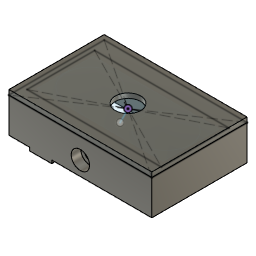
couvercle2_female (Autodesk Fusion 360 design; units mm, degrees)
Autodesk Fusion 360 part; units mm, degrees
sketch "Esquisse7" plane through (0, 0, 10) normal (0, 0, 1) x (-1, 0, 0)
  circle A0 centre (-12, 0) radius 7.6
  circle A1 centre (12, 0) radius 7.6
  line L0 (-19.9, -8.9) -> (19.9, -8.9)
  line L1 (19.9, -8.9) -> (19.9, 8.9)
  line L2 (19.9, 8.9) -> (-19.9, 8.9)
  line L3 (-19.9, 8.9) -> (-19.9, -8.9)
  line L4 (0, 0) -> (-2.53, 5.0152)
  constraint coincident L4.start origin
sketch "Esquisse3" plane through (0, 0, 10) normal (0, 0, 1) x (-1, 0, 0)
  line L0 (21.15, -10.65) -> (-21.15, -10.65)
  line L1 (-21.15, -10.65) -> (-21.15, 10.65)
  line L2 (-21.15, 10.65) -> (21.15, 10.65)
  line L3 (21.15, 10.65) -> (21.15, -10.65)
  line L4 (21.15, -10.65) -> (-21.15, 10.65) construction
  line L5 (-21.15, -10.65) -> (21.15, 10.65) construction
  line L6 (22.5, -15) -> (-22.5, -15)
  line L7 (-22.5, -15) -> (-22.5, 15)
  line L8 (-22.5, 15) -> (22.5, 15)
  line L9 (22.5, 15) -> (22.5, -15)
  line L10 (22.5, -15) -> (-22.5, 15) construction
  line L11 (-22.5, -15) -> (22.5, 15) construction
  dimension "d76" = 42.3
  dimension "d77" = 21.3
  dimension "d78" = 45
  dimension "d79" = 30
  constraint horizontal L0
  constraint perpendicular L0 L1
  constraint parallel L0 L2
  constraint parallel L1 L3
  constraint coincident L4 origin
  constraint coincident L5 origin
  constraint horizontal L6
  constraint perpendicular L6 L7
  constraint parallel L6 L8
  constraint parallel L7 L9
  constraint coincident L10 origin
  constraint coincident L11 origin
  measures "d76" distance of L1.end L2.end
  measures "d77" distance of L0.end L1.end
  measures "d78" distance of L7.end L8.end
  measures "d79" distance of L6.end L7.end
extrude "Extrusion1" add sketch "Esquisse3" against normal blind 11
extrude "Extrusion2" add sketch "Esquisse3" along normal blind 1.5 contours L0 L1 L2 L3 | L6 L7 L8 L9
sketch "Esquisse4" plane through (0, -15, 0) normal (0, -1, 0) x (1, 0, 0)
  line L0 (-22.5, 11.5) -> (-22.5, -1)
  line L1 (-22.5, -1) -> (22.5, -1)
  line L2 (22.5, -1) -> (22.5, 11.5)
  line L3 (22.5, 11.5) -> (-22.5, 11.5)
  line L4 (0, 0) -> (0, 3.5)
  dimension "d84" = 3.5
  constraint coincident L4.start origin
  constraint vertical L4
  measures "d84" distance of L4.start L4.end
hole "Perçage1" at (0, -15, 3.5) direction (0, 1, 0) diameter 3.3 depth 8 tip angle 180 counterbore diameter 5.8 counterbore depth 3
sketch "Esquisse5" plane through (0, 15, 0) normal (0, 1, 0) x (-1, 0, 0)
  line L0 (-22.5, 11.5) -> (-22.5, -1)
  line L1 (-22.5, -1) -> (22.5, -1)
  line L2 (22.5, -1) -> (22.5, 11.5)
  line L3 (22.5, 11.5) -> (-22.5, 11.5)
  line L4 (0, 0) -> (0, 3.5)
  dimension "d100" = 3.5
  constraint coincident L4.start origin
  constraint vertical L4
  measures "d100" distance of L4.start L4.end
hole "Perçage2" at (0, 15, 3.5) direction (0, -1, 0) diameter 3.3 depth 8 tip angle 180 counterbore diameter 5.8 counterbore depth 3
hole "Perçage3" at (0, 0, 11.5) direction (0, 0, -1) diameter 8 depth 1.5 tip angle 180
sketch "Esquisse6" plane through (0, 0, -1) normal (0, 0, -1) x (1, 0, 0)
  line L0 (-21.15, 10.65) -> (21.15, 10.65)
  line L1 (21.15, 10.65) -> (21.15, -10.65)
  line L2 (21.15, -10.65) -> (-21.15, -10.65)
  line L3 (-21.15, -10.65) -> (-21.15, 10.65)
  line L4 (22.5, 15) -> (-22.5, 15)
  line L5 (-22.5, 15) -> (-22.5, -15)
  line L6 (-22.5, -15) -> (22.5, -15)
  line L7 (22.5, -15) -> (22.5, 15)
  line L8 (-22.5, 15) -> (-12.5, 15)
  circle A0 centre (-12.5, 15) radius 3.5
  line L9 (22.5, -15) -> (12.5, -15)
  circle A1 centre (12.5, -15) radius 3.5
  dimension "d119" = 7
  dimension "d120" = 10
  dimension "d121" = 7
  constraint coincident L4.end L5.start
  constraint coincident L4 L8.end
  constraint perpendicular L5 L8
  constraint coincident L8.end A0.centre
  constraint coincident L6.end L7.start
  constraint perpendicular L7 L9
  constraint coincident L9.end A1.centre
  measures "d119" diameter of A0
  measures "d120" distance of L6.end L9.end
  measures "d121" diameter of A1
extrude "Extrusion3" add sketch "Esquisse6" along normal blind 1 contours L4 L8 A0 | L6 L9 A1 picked at (-14.8203, 14.8261) picked at (10.334, -14.1499)
